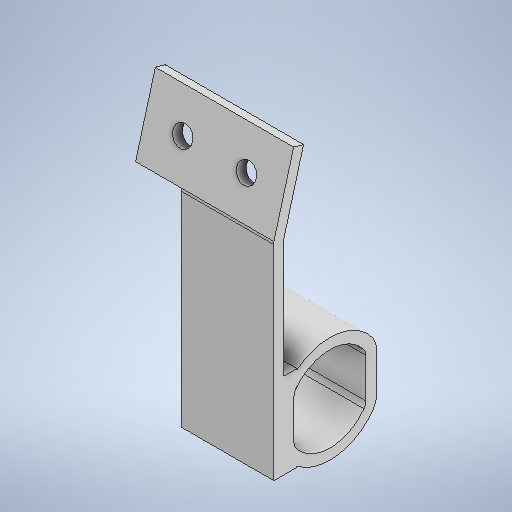
# Autodesk Inventor part: leftWheeler
Saved by Autodesk Inventor 2025.1 (Build 291241000, 241)
## iProperties
Created: 2025-06-15
Part Number: leftWheeler
Material: Generic
Document SubType Name: Modeling
Designer: User
Density: 1 g/cm^3
Appearance: Default
Author: User
## iProperties of the stored document leftWheeler_3DPrint.ipt
Created: 2025-06-15
Part Number: leftWheeler_3DPrint
Material: Generic
Document SubType Name: Modeling
Designer: User
Density: 1 g/cm^3
Appearance: Default
Author: User
Autodesk Inventor part; units mm, degrees
ref_plane "YZ Plane" through (0, 0, 0) normal (1, 0, 0) x (0, 1, 0)
ref_plane "XZ Plane" through (0, 0, 0) normal (0, 1, 0) x (-1, 0, 0)
sketch "Sketch1" plane through (0, 0, 0) normal (0, 0, 1) x (1, 0, 0)
  line L0 (1, 9) -> (14, 9) projected
  line L1 (1, 3) -> (1, 9) projected
  line L2 (14, 3) -> (1, 3) projected
  line L3 (14, 9) -> (14, 3) projected
  line L4 (1, 12) -> (14, 12)
  line L5 (1, 0) -> (14, 0)
  line L6 (1, 12.5) -> (14, 12.5)
  line L7 (1, -0.5) -> (14, -0.5)
  line L8 (0, 1.4) -> (0, 10.6) projected
  line L9 (0, -0.5) -> (14, -0.5)
  line L10 (14, -0.5) -> (14, 12.5)
  line L11 (14, 12.5) -> (0, 12.5)
  line L12 (0, 12.5) -> (0, -0.5)
  point P0 (0, 0)
  dimension "d0" = 0.5
  dimension "d1" = 0.5
  constraints: 16 end point, 4 parallel, 3 horizontal, 1 perpendicular, 4 other
  measures "d0" distance between parallel lines of L4 L6
  measures "d1" distance between parallel lines of L5 L7
extrude "Extrusion1" add sketch "Sketch1" along normal blind 2
sketch "Sketch2" plane through (14, -0.5, 0) normal (1, 0, 0) x (0, 0, -1)
  line L0 (10, 9.5) -> (10, 3.5) projected
  line L1 (10.5, 9.5) -> (10.5, 3.5)
  line L2 (0, 13) -> (0, 0) projected
  line L3 (0.0028, 13) -> (0, 0)
  arc A0 (5, 0.5) -> (9.8, 2.9) centre (5, 6.5) ccw projected
  spline S0 degree 3 poles (9.8, 10.1) (9.3822, 10.6561) (8.439, 11.5426) (6.738, 12.3306) (5.0002, 12.5848) (3.2616, 12.3308) (1.5615, 11.5422) (0.6175, 10.6564) (0.2, 10.1) knots 0.000048 0.000048 0.000048 0.000048 1.982593 3.634064 5.285536 6.937008 8.58848 10.571071 10.571071 10.571071 10.571071 weights 1 1 1 1 1 1 1 1 1 projected
  arc A1 (0.2, 2.9) -> (5, 0.5) centre (5, 6.5) ccw projected
  ellipse E0 centre (0.7683, 3.4229) end of major axis (0.4925, 4.2518) minor radius 0.7558 (0, 3.5) -> (0.2, 2.9) ccw projected
  ellipse E1 centre (0.7685, 9.5775) end of major axis (1.0457, 10.4061) minor radius 0.7558 (0.2, 10.1) -> (0, 9.5) ccw projected
  ellipse E2 centre (9.2317, 3.4229) end of major axis (9.5075, 4.2518) minor radius 0.7558 (9.8, 2.9) -> (10, 3.5) ccw projected
  ellipse E3 centre (9.2318, 9.5768) end of major axis (8.9568, 10.4058) minor radius 0.7558 (10, 9.5) -> (9.7999, 10.1) ccw projected
  arc A2 (5, 0.0295) -> (10.1758, 2.6168) centre (5, 6.5) ccw
  arc A3 (-0.1717, 2.6115) -> (5, 0.0295) centre (5, 6.5) ccw
  line L4 (10.4705, 3.4977) -> (10.4705, 9.5023)
  ellipse E4 centre (0.7683, 3.4229) end of major axis (0.3339, 4.718) minor radius 1.2242 (-0.4709, 3.5051) -> (-0.1717, 2.6115) ccw
  ellipse E5 centre (0.7685, 9.5775) end of major axis (1.1957, 10.8767) minor radius 1.2233 (-0.1748, 10.3845) -> (-0.4697, 9.4882) ccw
  arc A4 (0.2, 2.9) -> (9.8, 2.9) centre (5, 6.5) ccw projected
  arc A5 (5, -1.5631) -> (11.4481, 1.6589) centre (5, 6.5) ccw
  arc A6 (-1.4235, 1.6263) -> (5, -1.5631) centre (5, 6.5) ccw
  line L5 (12.0631, 3.4977) -> (12.0631, 9.5023)
  ellipse E6 centre (0.7683, 3.4229) end of major axis (-0.2657, 6.5587) minor radius 2.7801 (-2.0629, 3.5774) -> (-1.4235, 1.6263) ccw
  ellipse E7 centre (0.7685, 9.5775) end of major axis (1.7896, 12.7173) minor radius 2.7798 (-1.4322, 11.3622) -> (-2.0617, 9.4138) ccw
  line L6 (-0.4709, 3.5051) -> (-0.4697, 9.4882)
  line L7 (-2.0629, 3.5774) -> (-2.0617, 9.4138)
  spline S1 degree 5 poles (10.1762, 10.3826) (9.455, 11.3411) (8.5153, 12.1382) (7.3995, 12.6912) (5.0003, 13.2497) (2.6, 12.6917) (1.4857, 12.137) (0.5444, 11.3415) (-0.1764, 10.3824) knots 0 0 0 0 0 0 0.499984 0.499984 0.499984 1 1 1 1 1 1
  spline S2 degree 3 poles (10.1759, 2.6167) (10.3655, 2.8683) (10.4707, 3.1827) (10.4707, 3.4977) knots 0 0 0 0 1 1 1 1
  spline S3 degree 3 poles (10.4707, 9.5023) (10.4707, 9.8173) (10.3655, 10.1318) (10.1757, 10.3833) knots 0 0 0 0 1 1 1 1
  spline S4 degree 4 poles (11.4481, 1.6589) (11.7448, 2.0529) (11.9559, 2.5113) (12.0631, 3.0045) (12.0631, 3.4977) knots 0 0 0 0 0 1 1 1 1 1
  spline S5 degree 4 poles (12.0631, 9.5023) (12.0631, 9.995) (11.9561, 10.4877) (11.7455, 10.9457) (11.4492, 11.3395) knots 0 0 0 0 0 1 1 1 1 1
  spline S6 degree 5 poles (11.4495, 11.3391) (10.5511, 12.5335) (9.3795, 13.5256) (7.9898, 14.2154) (5.0062, 14.9093) (2.0215, 14.2187) (0.6377, 13.5325) (-0.5334, 12.5493) (-1.4322, 11.3622) knots 0 0 0 0 0 0 0.500955 0.500955 0.500955 1 1 1 1 1 1
  point P0 (0, 0.5)
  point P1 (0, 10.6069)
  point P2 (0, 12.8255)
  point P3 (0, 0.1744)
  point P4 (0, 2.393)
  point P5 (0.0005, 2.3924)
  point P6 (0, 0.1743)
  point P7 (0.0027, 12.8276)
  point P8 (0.0023, 10.6096)
  constraints: 12 end point, 8 point on circle, 7 parallel, 4 centre point, 41 other
extrude "Extrusion2" add sketch "Sketch2" along normal blind 2 contours L3 S6 S5 L5 S4 A5 A6 L2 A3 A2 S2 L4 S3 S1 | S1 E5 L6 E4 A3 L2 A6 E6 L7 E7 S6
sketch "Sketch3" plane through (14, 1.893, 0) normal (1, 0, 0) x (0, 0, -1)
  arc A0 (-0.1717, 0.2185) -> (0, 0) centre (5, 4.107) ccw projected
  line L0 (0, 0) -> (0, 8.2139) projected
  arc A1 (0, 8.2139) -> (-0.1748, 7.9915) centre (4.9785, 4.1209) ccw projected
  ellipse E0 centre (0.7685, 7.1845) end of major axis (0.3413, 5.8853) minor radius 1.2233 (-0.1748, 7.9915) -> (-0.4697, 7.0952) ccw projected
  line L1 (-0.4697, 7.0952) -> (-0.4709, 1.1121) projected
  ellipse E1 centre (0.7683, 1.03) end of major axis (1.2028, -0.2651) minor radius 1.2242 (-0.4709, 1.1121) -> (-0.1717, 0.2185) ccw projected
  point P0 (0, -1.893)
  constraints: 2 other
extrude "Extrusion3" cut sketch "Sketch3" against normal through all
sketch "Sketch4" plane through (14, -0.5, 0) normal (-1, 0, 0) x (0, 0, 1)
  line L0 (-10.4705, 9.5023) -> (-10.4705, 3.4977) projected
  ellipse E0 centre (-9.2512, 9.5832) end of major axis (-8.8307, 10.8511) minor radius 1.2058 (-10.1756, 10.3833) -> (-10.4705, 9.5023) ccw projected
  spline S0 degree 5 poles (-0.0023, 10.6096) (-0.7281, 11.4914) (-1.6474, 12.2152) (-2.7157, 12.7179) (-5.0579, 13.2362) (-7.3991, 12.6912) (-8.5148, 12.1385) (-9.4545, 11.3415) (-10.1756, 10.3833) knots 0 0 0 0 0 0 0.487709 0.487709 0.487709 1 1 1 1 1 1 projected
  line L1 (-0.0027, 12.8276) -> (-0.0023, 10.6096) projected
  spline S1 degree 5 poles (-11.4492, 11.3395) (-10.5511, 12.5335) (-9.3795, 13.5256) (-7.9898, 14.2154) (-5.4174, 14.8137) (-2.8441, 14.3827) (-1.8061, 14.0228) (-0.8486, 13.496) (-0.0027, 12.8277) knots 0 0 0 0 0 0 0.581033 0.581033 0.581033 1 1 1 1 1 1 projected
  ellipse E1 centre (-9.2769, 9.5918) end of major axis (-8.3583, 12.3614) minor radius 2.7713 (-11.4492, 11.3395) -> (-12.0631, 9.5023) ccw projected
  line L2 (-12.0631, 3.4977) -> (-12.0631, 9.5023) projected
  ellipse E2 centre (-9.2769, 3.4079) end of major axis (-10.1984, 6.1767) minor radius 2.7712 (-12.0631, 3.4977) -> (-11.4481, 1.6589) ccw projected
  arc A0 (-11.4481, 1.6589) -> (0, 0.1743) centre (-5, 6.5) ccw projected
  line L3 (-0.0005, 2.3924) -> (0, 0.1743) projected
  arc A1 (-10.1758, 2.6168) -> (-0.0005, 2.3924) centre (-5, 6.5) ccw projected
  ellipse E3 centre (-9.2512, 3.4164) end of major axis (-9.673, 4.684) minor radius 1.2058 (-10.4705, 3.4977) -> (-10.1758, 2.6168) ccw projected
  point P0 (0, 0.5)
  constraints: 6 other
extrude "Extrusion4" add sketch "Sketch4" along normal up to surface (14 mm away)
sketch "Sketch5" plane through (0, -0.5, 0) normal (0, -1, 0) x (1, 0, 0)
  line L0 (0, 2) -> (14, 2) projected
  line L1 (0, 2) -> (14, 2)
  line L2 (14, 2) -> (14, 3.5)
  line L3 (14, 3.5) -> (0, 3.5)
  line L4 (0, 3.5) -> (0, 2)
  point P0 (0, 0)
  dimension "d22" = 1.5
  constraints: 8 end point, 2 parallel, 1 horizontal, 1 perpendicular
  measures "d22" distance of L2.end L1.end
ref_plane "Work Plane1" through (-71.4012, 38.5222, -12.5) normal (0.0153412, 0.9998823, 0) x (0, 0, 1)
extrude "Extrusion5" add sketch "Sketch5" against normal up to surface surface through (-71.4012, 38.5222, -12.5) normal (0.0153412, 0.9998823, 0)
sketch "Sketch6" plane through (0, -0.5, 3.5) normal (0, 0, 1) x (1, 0, 0)
  line L0 (14, 0) -> (14, 37.7119) projected
  line L1 (14, 37.7119) -> (0, 37.9267) projected
  line L2 (-54.2389, 27.7576) -> (-67.6625, 27.9635) projected
  line L3 (14, 37.7119) -> (14, 26.7106)
  line L4 (14, 13) -> (14, 37.7119) projected
  line L5 (14, 26.7106) -> (-6.9975, 27.0328)
  line L6 (14, 37.7119) -> (-6.9975, 38.034)
  line L7 (-6.9975, 38.034) -> (-6.9975, 27.0328)
  point P0 (0, 0.5)
  point P1 (4.9084, 26.8501)
  dimension "d25" = 21
  dimension "d26" = 21
  constraints: 8 end point, 3 point on line
  measures "d25" distance of L3.end L5.end
  measures "d26" distance of L0.end L6.end
extrude "Extrusion6" add sketch "Sketch6" against normal blind 1.5
sketch "Sketch7" plane through (0, -0.5, 3.5) normal (0, 0, 1) x (1, 0, 0)
  line L0 (14, 0) -> (14, 37.7119) projected
  line L1 (14, -3.9463) -> (21.7341, -3.9463)
  line L2 (21.7341, -3.9463) -> (21.7341, 19.3789)
  line L3 (21.7341, 19.3789) -> (14, 19.3789)
  line L4 (14, 19.3789) -> (14, -3.9463)
  point P0 (0, 0.5)
  constraints: 8 end point, 2 parallel, 1 horizontal, 1 perpendicular
extrude "Extrusion7" cut sketch "Sketch7" against normal blind 15.75
sketch "Sketch8" plane through (14, 10.1069, 0) normal (1, 0, 0) x (0, 0, -1)
  ellipse E0 centre (9.2512, -1.0236) end of major axis (8.8307, 0.2442) minor radius 1.2058 (10.4705, -1.1046) -> (10.1756, -0.2236) ccw projected
  line L0 (10.4705, -7.1091) -> (10.4705, -1.1046) projected
  ellipse E1 centre (9.2512, -7.1904) end of major axis (9.673, -5.9229) minor radius 1.2058 (10.1758, -7.9901) -> (10.4705, -7.1091) ccw projected
  arc A0 (0.0005, -8.2145) -> (10.1758, -7.9901) centre (5, -4.1069) ccw projected
  line L1 (0, -10.4326) -> (0.0005, -8.2145) projected
  arc A1 (0, -10.4326) -> (11.4481, -8.948) centre (5, -4.1069) ccw projected
  ellipse E2 centre (9.2769, -7.199) end of major axis (10.1984, -4.4302) minor radius 2.7712 (11.4481, -8.948) -> (12.0631, -7.1091) ccw projected
  line L2 (12.0631, -1.1046) -> (12.0631, -7.1091) projected
  ellipse E3 centre (9.2769, -1.0151) end of major axis (8.3583, 1.7545) minor radius 2.7713 (12.0631, -1.1046) -> (11.4492, 0.7326) ccw projected
  spline S0 degree 5 poles (0.0027, 2.2208) (0.8486, 2.8891) (1.8061, 3.4159) (2.8441, 3.7759) (5.4174, 4.2068) (7.9898, 3.6085) (9.3795, 2.9188) (10.5511, 1.9266) (11.4492, 0.7326) knots 0 0 0 0 0 0 0.418967 0.418967 0.418967 1 1 1 1 1 1 projected
  line L3 (0.0023, 0.0028) -> (0.0027, 2.2208) projected
  spline S1 degree 5 poles (10.1756, -0.2236) (9.4545, 0.7346) (8.5148, 1.5316) (7.3991, 2.0844) (5.0579, 2.6294) (2.7157, 2.111) (1.6474, 1.6084) (0.7281, 0.8845) (0.0023, 0.0027) knots 0 0 0 0 0 0 0.512291 0.512291 0.512291 1 1 1 1 1 1 projected
  arc A2 (-0.1717, -7.9954) -> (0, -8.2139) centre (5, -4.1069) ccw projected
  ellipse E4 centre (0.7683, -7.184) end of major axis (1.2028, -8.479) minor radius 1.2242 (-0.4709, -7.1018) -> (-0.1717, -7.9954) ccw projected
  ellipse E5 centre (0.7685, -1.0294) end of major axis (0.3413, -2.3286) minor radius 1.2233 (-0.1748, -0.2224) -> (-0.4697, -1.1187) ccw projected
  arc A3 (0, 0) -> (-0.1748, -0.2224) centre (4.9785, -4.093) ccw projected
  line L4 (-0.4697, -1.1187) -> (-0.4709, -7.1018) projected
  line L5 (0, 0) -> (0, 2.3931) projected
  line L6 (0, 2.3931) -> (-2, 2.3931) projected
  line L7 (0, -10.6069) -> (0, -8.2139) projected
  line L8 (0, -10.6069) -> (-3.5, -10.6069) projected
  line L9 (1.2443, -11.2419) -> (1.2443, -9.3759)
  arc A4 (0.0005, -8.2145) -> (10.1758, -7.9901) centre (5, -4.1069) ccw projected
  arc A5 (0.0005, -8.2145) -> (1.2443, -9.3759) centre (4.9979, -4.1091) ccw
  line L10 (0, -8.2139) -> (-0.1717, -7.9954)
  ellipse E6 centre (0.7683, -7.184) end of major axis (1.2028, -8.479) minor radius 1.2242 (-0.4709, -7.1018) -> (-0.1717, -7.9954) ccw projected
  line L11 (-0.1717, -7.9954) -> (-0.1717, -10.6069)
  line L12 (0, -10.6069) -> (-0.1717, -10.6069)
  line L13 (0, -10.6069) -> (0, -10.4326)
  arc A6 (0, -10.4326) -> (1.2443, -11.2419) centre (5, -4.1069) ccw
  line L14 (1.2444, 1.1622) -> (1.2444, 3.0282)
  arc A7 (1.2444, 3.0282) -> (0.0027, 2.2208) centre (4.9892, -4.0883) ccw
  line L15 (0, 2.3931) -> (0, 0) projected
  line L16 (0.0027, 2.2208) -> (0, 2.3931)
  line L17 (0, 2.3931) -> (-0.1717, 2.3931)
  line L18 (-0.1717, 2.3931) -> (-0.1748, -0.2224)
  line L19 (-0.1748, -0.2224) -> (0.0023, 0.0028)
  line L20 (0.0005, -8.2145) -> (0, -8.2139)
  point P0 (0, -10.1069)
  constraints: 22 end point, 9 point on circle, 3 centre point, 2 perpendicular, 2 point on line, 2 tangent, 2 vertical, 13 other
extrude "Extrusion8" add sketch "Sketch8" against normal up to surface (14 mm away) contours S1 L3 S0 L14 | L19 L5 L16 L3 | L9 A1 L1 A0 | A3 L18 L6 L5 | L1 L7 L8 L11 A2
sketch "Sketch9" plane through (0, -0.5, 3.5) normal (0, 0, 1) x (1, 0, 0)
  line L0 (0, 0) -> (0, 26.9254) projected
  line L1 (14, 0) -> (0, 0) projected
  line L2 (14, 0) -> (14, 37.7119) projected
  line L3 (14, 37.7119) -> (-6.9975, 38.034) projected
  line L4 (-6.9975, 38.034) -> (-6.9975, 27.0328) projected
  line L5 (-6.9975, 27.0328) -> (0, 26.9254) projected
  line L6 (-6.9975, 38.034) -> (14, 37.7119) projected
  line L7 (-6.9975, 38.034) -> (14, 26.7132)
  line L8 (14, 13) -> (14, 37.7119) projected
  line L9 (14, 37.7119) -> (-6.9975, 27.0328)
  line L10 (-6.9975, 38.034) -> (-6.9975, 27.0328) projected
  line L11 (-6.9975, 32.3723) -> (14, 32.3723)
  line L12 (-6.9975, 32.3723) -> (0.0025, 32.3723)
  line L13 (14, 32.3723) -> (7, 32.3723)
  line L14 (-6.9975, 32.3723) -> (-1.9975, 32.3723)
  line L15 (14, 32.3723) -> (9, 32.3723)
  circle A0 centre (-1.9975, 32.3723) radius 1.5
  circle A1 centre (9, 32.3723) radius 1.5
  point P0 (0, 0.5)
  dimension "d35" = 5
  dimension "d36" = 5
  dimension "d37" = 3
  dimension "d38" = 3
  constraints: 14 end point, 7 point on line, 2 centre point, 2 coincident, 1 perpendicular
  measures "d35" distance of L11.start L14.end
  measures "d36" distance of L11.end L15.end
  measures "d37" diameter of A0
  measures "d38" diameter of A1
extrude "Extrusion9" cut sketch "Sketch9" against normal blind 3 contours A0 L11 | L11 A0 | A1 L11 | L11 A1
sketch "Sketch10" plane through (14, 2.9977, -12.0631) normal (1, 0, 0) x (0, 0, -1)
  line L0 (-12.0631, 9.5023) -> (-14.0631, 9.5023) projected
  line L1 (-15.5631, -3.4977) -> (-15.5631, 34.2141) projected
  line L2 (-15.5631, 23.535) -> (-15.5631, 23.4276) projected
  line L3 (-15.5631, 23.535) -> (-14.0631, 23.535) projected
  line L4 (-14.0631, 9.5023) -> (-14.0631, 34.2141) projected
  line L5 (-14.0631, 34.2141) -> (-15.5631, 34.2141) projected
  line L6 (-15.5631, 34.2141) -> (-12.5631, 34.2141)
  line L7 (-14.0631, 34.2141) -> (-11.0631, 34.2141)
  line L8 (-14.0631, 23.535) -> (-11.0631, 34.2141)
  line L9 (-11.0631, 34.2141) -> (-12.5072, 34.6198)
  line L10 (-12.5072, 34.6198) -> (-15.5631, 23.535)
  point P0 (-12.0631, -2.9977)
  point P1 (-12.6191, 34.2141)
  point P2 (-14.0631, 28.976)
  point P3 (-12.5631, 34.2141)
  dimension "d41" = 3
  dimension "d42" = 3
  dimension "d43" = 1.5
  constraints: 10 end point, 1 horizontal, 1 perpendicular, 1 point on line
  measures "d41" distance of L1.end L6.end
  measures "d42" distance of L4.end L7.end
  measures "d43" distance of L7.end L9.end
extrude "Extrusion10" add sketch "Sketch10" against normal up to surface (20.9975 mm away) contours L4 L10 L6 L7 L8
sketch "Sketch11" plane through (14, 2.9977, -12.0631) normal (1, 0, 0) x (0, 0, -1)
  line L0 (-15.5631, -3.4977) -> (-15.5631, 34.2141) projected
  line L1 (-14.0631, 28.976) -> (-14.0631, 34.2141) projected
  line L2 (-15.5631, 34.5363) -> (-14.0631, 34.5363) projected
  line L3 (-15.5631, 34.2141) -> (-15.5631, 34.5363) projected
  line L4 (-14.0631, 34.5363) -> (-14.0631, 34.2141) projected
  line L5 (-12.6191, 34.2141) -> (-14.0631, 28.976) projected
  line L6 (-15.5631, 23.535) -> (-14.0631, 23.535) projected
  line L7 (-12.6191, 34.2141) -> (-15.5631, 23.535)
  point P0 (-12.0631, -2.9977)
  point P1 (-14.0631, 28.976)
  constraints: 2 end point
extrude "Extrusion11" cut sketch "Sketch11" against normal through all
sketch "Sketch12" plane through (-6.9975, 26.5328, 3.5) normal (0, 0.2657691, 0.9640367) x (1, 0, 0)
  ellipse E0 centre (15.9975, 5.5388) end of major axis (15.9975, 3.9828) minor radius 1.5 (14.501, 5.644) -> (17.4941, 5.644) ccw projected
  ellipse E1 centre (5, 5.5388) end of major axis (5, 3.9828) minor radius 1.5 (3.5034, 5.644) -> (6.4966, 5.644) ccw projected
  line L0 (17.4941, 5.644) -> (14.501, 5.644) projected
  line L1 (6.4966, 5.644) -> (3.5034, 5.644) projected
  point P0 (6.9975, -24.6484)
  constraints: 2 other
extrude "Extrusion12" add sketch "Sketch12" against normal up to surface surface through (14, 37.2119, -1) normal (0, -0.2704527, -0.9627333)
sketch "Sketch13" plane through (-6.9975, 26.5328, 3.5) normal (0, 0.2657691, 0.9640367) x (1, 0, 0)
  line L0 (0, 0.3987) -> (20.9975, 0.3987) projected
  line L1 (20.9975, 11.0775) -> (20.9975, 0) projected
  line L2 (20.9975, 11.0775) -> (0, 11.0775) projected
  line L3 (0, 0) -> (0, 11.0775) projected
  circle A0 centre (15.6581, 5.7381) radius 5.3394
  circle A1 centre (5.3394, 5.7381) radius 5.3394
  circle A2 centre (15.6581, 5.7381) radius 1.5
  circle A3 centre (5.3394, 5.7381) radius 1.5
  point P0 (6.9975, -24.6484)
  dimension "d50" = 3
  dimension "d51" = 3
  constraints: 6 tangent, 4 centre point, 2 coincident
  measures "d50" diameter of A2
  measures "d51" diameter of A3
extrude "Extrusion13" cut sketch "Sketch13" against normal through all contours A2 | A3
sketch "Sketch14" plane through (14, 2.9977, -12.0631) normal (1, 0, 0) x (0, 0, -1)
  line L0 (-12.6191, 34.2141) -> (-15.5631, 23.535) projected
  line L1 (-14.0631, 23.535) -> (-11.0631, 34.2141) projected
  line L2 (-11.0631, 34.2141) -> (-12.6191, 34.2141) projected
  line L3 (-15.5631, -3.4977) -> (-15.5631, 23.535) projected
  line L4 (-15.5631, 23.535) -> (-14.0631, 23.535)
  point P0 (-12.0631, -2.9977)
  constraints: 2 end point, 1 perpendicular
extrude "Extrusion14" cut sketch "Sketch14" against normal through all
sketch "Sketch15" plane through (0, 2.9977, -12.0631) normal (-1, 0, 0) x (0, 0, 1)
  line L0 (15.5631, 23.4276) -> (14.0631, 23.4276) projected
  line L1 (15.5631, 23.535) -> (15.5631, 23.4276) projected
  line L2 (15.5631, 23.535) -> (14.0631, 23.535) projected
  line L3 (14.0631, 23.4276) -> (14.0631, 23.535) projected
  point P0 (12.0631, -2.9977)
extrude "Extrusion15" cut sketch "Sketch15" along normal blind 10
sketch "Sketch17" plane through (14, 26.5328, 3.5) normal (0, 1, 0) x (1, 0, 0)
  line L0 (-14, 1.5) -> (-14, 0) projected
  line L1 (0, 0) -> (-14, 0) projected
  line L2 (0, 1.5) -> (0, 0) projected
  line L3 (-14, 1.5) -> (0, 1.5) projected
  point P0 (-14, 3.5)
extrude "Extrusion16" add sketch "Sketch17" along normal blind 4
sketch "Sketch18" plane through (14, 2.9977, -12.0631) normal (1, 0, 0) x (0, 0, -1)
  line L0 (-15.5631, 27.535) -> (-14.0631, 27.535) projected
  line L1 (-14.0631, 9.5023) -> (-14.0631, 27.535) projected
  line L2 (-14.0631, 27.535) -> (-11.0631, 27.535)
  line L3 (-14.0631, 27.535) -> (-11.0631, 38.4502)
  line L4 (-15.5631, -3.4977) -> (-15.5631, 27.535) projected
  line L5 (-15.5631, 27.535) -> (-15.5631, 27.9473)
  line L6 (-15.5631, 27.9473) -> (-12.5631, 38.8625)
  line L7 (-12.5631, 38.8625) -> (-11.0631, 38.4502)
  point P0 (-12.0631, -2.9977)
  dimension "d60" = 3
  dimension "d61" = 11.32
  constraints: 10 end point, 1 horizontal, 1 perpendicular, 1 vertical
  measures "d60" distance of L0.end L2.end
  measures "d61" distance of L0.end L3.end
extrude "Extrusion17" add sketch "Sketch18" against normal up to surface (14 mm away)
sketch "Sketch19" plane through (0, 2.9977, -12.0631) normal (-1, 0, 0) x (0, 0, 1)
  line L0 (14.0631, 27.535) -> (11.0631, 38.4502) projected
  line L1 (11.0631, 38.4502) -> (12.5631, 38.8625) projected
  line L2 (12.5631, 38.8625) -> (15.5631, 27.9473) projected
  line L3 (14.0631, 27.535) -> (15.5631, 27.9473)
  point P0 (12.0631, -2.9977)
  constraints: 2 end point
extrude "Extrusion18" add sketch "Sketch19" along normal blind 7
sketch "Sketch20" plane through (-7, 41.8603, 0.5) normal (0, 0.2650177, 0.9642436) x (1, 0, 0)
  line L0 (21, -11.32) -> (7, -11.32) projected
  line L1 (21, 0) -> (21, -11.32) projected
  line L2 (21, 0) -> (0, 0) projected
  line L3 (0, -11.32) -> (0, 0) projected
  line L4 (7, -11.32) -> (0, -11.32) projected
  circle A0 centre (5.66, -5.66) radius 5.66
  circle A1 centre (15.34, -5.66) radius 5.66
  circle A2 centre (15.34, -5.66) radius 1.5
  circle A3 centre (5.66, -5.66) radius 1.5
  point P0 (7, -40.231)
  dimension "d66" = 3
  dimension "d67" = 3
  constraints: 6 tangent, 4 centre point, 2 coincident
  measures "d66" diameter of A2
  measures "d67" diameter of A3
extrude "Extrusion19" cut sketch "Sketch20" against normal blind 7 contours A2 | A3
equation "\"d39\" = d37"
body "Solid1"
